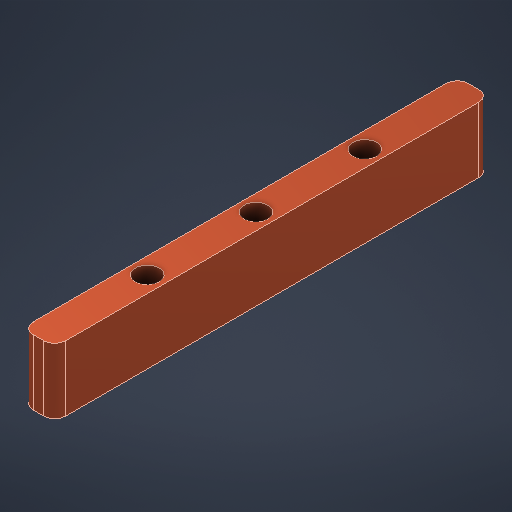
# Autodesk Inventor part: Bush
Saved by Autodesk Inventor 2026.2 (Build 302298000, 298)
## iProperties
Created: 2026-02-11
Part Number: Bush
Material: Медь
Document SubType Name: Modeling
Designer: EV-TECH
Density: 8.94 g/cm^3
Appearance: Медь — сатинированная
Author: EV-TECH
Autodesk Inventor part; units mm, degrees
ref_plane "YZ Plane" through (0, 0, 0) normal (1, 0, 0) x (0, 1, 0)
ref_plane "XZ Plane" through (0, 0, 0) normal (0, 1, 0) x (-1, 0, 0)
ref_plane "XY Plane" through (0, 0, 0) normal (0, 0, 1) x (1, 0, 0)
sketch "Эскиз1" plane through (0, 0, 0) normal (0, 1, 0) x (-1, 0, 0)
  line L0 (0, 0) -> (3, 0)
  line L1 (3, 0) -> (3, -40)
  line L2 (3, -40) -> (0, -40)
  line L3 (0, -40) -> (0, 0)
  line L4 (0, 0) -> (1, 0)
  line L5 (0, -5) -> (0, 0)
  line L6 (3, -40) -> (2, -40)
  line L7 (3, -35) -> (3, -40)
  dimension "d0" = 40
  dimension "d1" = 3
  constraints: 16 end point, 3 horizontal, 2 parallel, 1 perpendicular
  measures "d0" distance of L0.end L1.end
  measures "d1" distance of L0.start L0.end
extrude "Выдавливание1" add sketch "Эскиз1" along normal blind 6
sketch "Эскиз2" plane through (0, 0, 0) normal (0, -1, 0) x (1, 0, 0)
  line L0 (-3, 0) -> (0, 0) projected
  line L1 (-3, 0) -> (-2, 0)
  line L2 (-2, -5) -> (-1, -5)
  line L3 (-1, -5) -> (-1, -35)
  line L4 (-1, -35) -> (-2, -35)
  line L5 (-2, -35) -> (-2, -5)
  point P0 (0, -40)
  dimension "d13" = 30
  dimension "d14" = 1
  constraints: 10 end point, 2 horizontal, 2 parallel, 1 perpendicular
  measures "d13" distance of L4.end L2.start
  measures "d14" distance of L3.end L4.end
extrude "Выдавливание2" add sketch "Эскиз2" along normal blind 1
fillet "Сопряжение1" radius 1 4 edges at (0, 3, 0) (-3, 3, 0) (0, 3, -40) (-3, 3, -40)
fillet "Сопряжение2" radius 0.3 4 edges at (-1, -0.5, -35) (-2, -0.5, -35) (-1, -0.5, -5) (-2, -0.5, -5)
sketch "Эскиз3" plane through (0, 6, 0) normal (0, 1, 0) x (1, 0, 0)
  line L0 (0, 0) -> (-1.5, 0)
  line L1 (0, 1) -> (0, 39) projected
  line L2 (0, 20) -> (0, 30)
  circle A0 centre (-1.5, 10) radius 1.1
  circle A1 centre (-1.5, 20) radius 1.1
  circle A2 centre (-1.5, 30) radius 1.1
  dimension "d23" = 2.2
  dimension "d24" = 2.2
  dimension "d25" = 2.2
  constraints: 4 end point, 3 centre point, 1 horizontal, 1 point on line
  measures "d23" diameter of A0
  measures "d24" diameter of A1
  measures "d25" diameter of A2
extrude "Выдавливание3" cut sketch "Эскиз3" against normal blind 4
